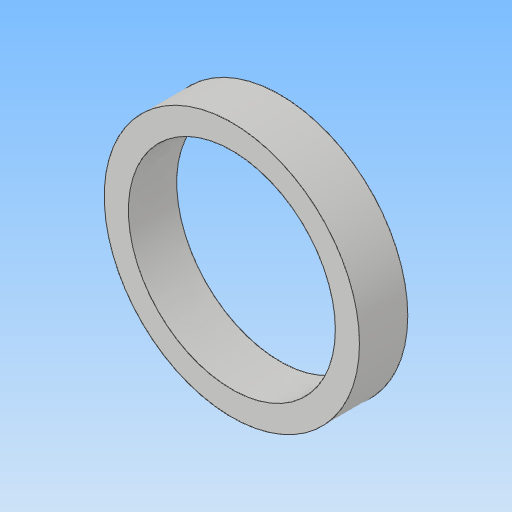
# Autodesk Inventor part: 45x58x7 bearing
Saved by Autodesk Inventor 2020.2 (Build 242310000, 310)
## iProperties
Created: 2016-11-19
Part Number: 45x58x7 bearing
Material: Allgemein
Document SubType Name: Modeling
Designer: paulg
Density: 1 g/cm^3
Appearance: Vorgabe
Author: paulg
Autodesk Inventor part; units mm, degrees
ref_plane "YZ Plane" through (0, 0, 0) normal (1, 0, 0) x (0, 1, 0)
ref_plane "XZ Plane" through (0, 0, 0) normal (0, 1, 0) x (-1, 0, 0)
ref_plane "XY Plane" through (0, 0, 0) normal (0, 0, 1) x (1, 0, 0)
sketch "Sketch1" plane through (0, 0, 0) normal (0, 0, 1) x (1, 0, 0)
  circle A0 centre (0, 0) radius 15
  circle A1 centre (0, 0) radius 18.5
  dimension "d4" = 15
  dimension "d6" = 18.5
  constraints: 2 centre point, 2 coincident
  measures "d4" radius of A0
  measures "d6" radius of A1
extrude "Extrusion1" add sketch "Sketch1" along normal blind 7
equation "\"d4\" = Rli"
equation "\"d6\" = Rla"
equation "\"E_\" = 1"
equation "\"Rr_\" = 2"
equation "\"R_\" = 19"
equation "\"Ri\" = 11.75"
equation "\"Rl\" = 17.5"
equation "\"Ra\" = 21.5"
equation "\"Rla\" = 18.5"
equation "\"Rli\" = 15"
equation "\"Rca\" = 7"
equation "\"Rea\" = 3.5"
equation "\"Rci\" = 5"
equation "\"Rei\" = 2"
equation "\"Ras\" = 1"
equation "\"Rsi\" = 5"
equation "\"Rsa\" = 7.5"
body "Solid1"
